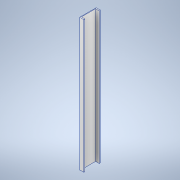
# Autodesk Inventor part: 14in-slide-pt_1
Saved by Autodesk Inventor 2020.1 (Build 241239000, 239)
## iProperties
Created: 2019-09-13
Part Number: 14in-slide-pt_1
Material: Aluminum 6061
Document SubType Name: Modeling
Designer: alpha
Density: 2.7 g/cm^3
Appearance: Aluminum - Flat
Author: alpha
Autodesk Inventor part; units mm, degrees
ref_plane "YZ Plane" through (0, 0, 0) normal (1, 0, 0) x (0, 1, 0)
ref_plane "XZ Plane" through (0, 0, 0) normal (0, 1, 0) x (-1, 0, 0)
ref_plane "XY Plane" through (0, 0, 0) normal (0, 0, 1) x (1, 0, 0)
sketch "Sketch2" plane through (0, 0, 0) normal (0, 1, 0) x (-1, 0, 0)
  line L0 (-5.5563, -22.225) -> (5.5563, -22.225)
  line L1 (5.5563, -22.225) -> (5.5563, 22.225)
  line L2 (5.5563, 22.225) -> (-5.5563, 22.225)
  line L3 (-5.5563, -22.225) -> (5.5563, 22.225) construction
  line L4 (5.5563, -22.225) -> (-5.5563, 22.225) construction
  line L5 (-11.1125, -19.05) -> (1.5875, 19.05) construction
  line L6 (1.5875, -19.05) -> (-11.1125, 19.05) construction
  line L7 (-5.5563, 19.05) -> (-5.5563, 22.225)
  line L8 (-5.5563, -19.05) -> (-5.5563, -22.225)
  line L9 (-5.5563, 19.05) -> (3.9688, 19.05)
  line L10 (3.9688, 19.05) -> (3.9687, -19.05)
  line L11 (3.9687, -19.05) -> (-5.5563, -19.05)
  point P0 (0, 0)
  point P1 (-4.7625, 0)
  dimension "d0" = 11.1125
  dimension "d1" = 44.45
  dimension "d6" = 9.525
  dimension "d7" = 90
  constraints: 24 end point, 4 midpoint, 3 horizontal, 2 vertical, 1 parallel, 1 perpendicular
  measures "d0" distance of L2.end L1.end
  measures "d1" distance of L1.end L0.end
  measures "d6" distance of L7.start L9.end
  measures "d7" angle of L9 L10
extrude "Extrusion1" add sketch "Sketch2" along normal blind 355.6
body "Solid1"
